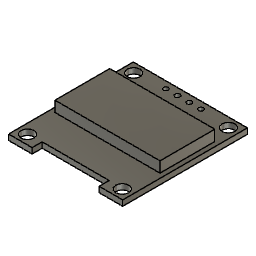
SSD1306 v2 (Autodesk Fusion 360 design; units mm, degrees)
Autodesk Fusion 360 part; units mm, degrees
note: some values were not read from the file. Set by a fixed rule: which sketch regions a step uses.
sketch "Sketch1" plane through (0, 0, 0) normal (0, 0, 1) x (1, 0, 0)
  line L0 (-12.35, 13.5) -> (12.35, 13.5)
  line L1 (12.35, 13.5) -> (12.35, -13.5)
  line L2 (-12.35, -13.5) -> (-12.35, 13.5)
  line L3 (0, 13.5) -> (0, -13.5)
  line L4 (-12.35, 0) -> (12.35, 0)
  circle A0 centre (-10.25, 11.5) radius 1.4
  circle A1 centre (10.25, 11.5) radius 1.4
  circle A2 centre (-10.25, -11.5) radius 1.4
  circle A3 centre (10.25, -11.5) radius 1.4
  line L5 (-7.2537, -13.5) -> (-7.2537, -11.3301)
  line L6 (-7.2537, -11.3301) -> (7.2537, -11.3301)
  line L7 (7.2537, -11.3301) -> (7.2537, -13.5)
  line L8 (7.2537, -13.5) -> (12.35, -13.5)
  line L9 (-12.35, -13.5) -> (-7.2537, -13.5)
  dimension "d1" = 24.7
  dimension "d2" = 27
  dimension "d11" = 2.8
  dimension "d12" = 2
  dimension "d13" = 2.1
  dimension "d15" = 23
  constraint horizontal L0
  constraint vertical L1
  constraint vertical L2
  constraint midpoint L0 L3.start
  constraint midpoint L2 L4.start
  constraint midpoint L1 L4.end
  constraint midpoint L4 origin
  constraint symmetric L3 A0 A1
  constraint symmetric L3 A2 A3
  constraint equal A0 A2
  constraint vertical A0.centre A2.centre
  constraint perpendicular L3 L6
  constraint symmetric L3 L5 L7
  constraint perpendicular L1 L8
  constraint perpendicular L5 L9
  measures "d1" distance of L0.start L0.end
  measures "d2" distance of L0.end L1.end
  measures "d11" diameter of A1
  measures "d12" distance of L0 A0.centre
  measures "d13" distance of L2 A0.centre
  measures "d15" distance of A0.centre A2.centre
extrude "Extrude2" add sketch "Sketch1" along normal blind 1.2 makes body 1
sketch "Sketch3" plane through (0, 0, 1.2) normal (0, 0, 1) x (-1, 0, 0)
  circle A0 centre (10.25, -11.5) radius 1.4
  circle A1 centre (-10.25, -11.5) radius 1.4
  circle A2 centre (-10.25, 11.5) radius 1.4
  circle A3 centre (10.25, 11.5) radius 1.4
  line L0 (-12.35, 13.5) -> (-12.35, -13.5)
  line L1 (-12.35, -13.5) -> (12.35, -13.5)
  line L2 (12.35, -13.5) -> (12.35, 13.5)
  line L3 (11.37, -7.42) -> (-11.37, -7.42)
  line L4 (-11.37, -7.42) -> (-11.37, 4.44)
  line L5 (-11.37, 4.44) -> (11.37, 4.44)
  line L6 (11.37, 4.44) -> (11.37, -7.42)
  line L7 (0, -13.5) -> (0, 13.5)
  line L8 (12.35, -13.5) -> (-12.35, -13.5)
  line L9 (12.35, 13.5) -> (7.2537, 13.5)
  line L10 (7.2537, 13.5) -> (7.2537, 11.3301)
  line L11 (7.2537, 11.3301) -> (-7.2537, 11.3301)
  line L12 (-7.2537, 11.3301) -> (-7.2537, 13.5)
  line L13 (-7.2537, 13.5) -> (-12.35, 13.5)
  dimension "d18" = 22.74
  dimension "d19" = 11.86
  dimension "d20" = 6.08
  constraint horizontal L3
  constraint vertical L4
  constraint horizontal L5
  constraint vertical L6
  constraint symmetric L4 L6 L7
  measures "d18" distance of L3.start L3.end
  measures "d19" distance of L3.start L5.end
  measures "d20" distance of L3 L8
extrude "Extrude3" add sketch "Sketch3" along normal blind 2.3 separate body contours L3 L5 L6 L7 | L3 L4 L5 L7 makes body 2
sketch "Sketch4" plane through (0, 0, 1.2) normal (0, 0, 1) x (-1, 0, 0)
  circle A0 centre (10.25, -11.5) radius 1.4
  circle A1 centre (-10.25, -11.5) radius 1.4
  circle A2 centre (10.25, 11.5) radius 1.4
  circle A3 centre (-10.25, 11.5) radius 1.4
  line L0 (12.35, -13.5) -> (12.35, 13.5)
  line L1 (12.35, 13.5) -> (7.2537, 13.5)
  line L2 (7.2537, 13.5) -> (7.2537, 11.3301)
  line L3 (7.2537, 11.3301) -> (-7.2537, 11.3301)
  line L4 (-7.2537, 11.3301) -> (-7.2537, 13.5)
  line L5 (-7.2537, 13.5) -> (-12.35, 13.5)
  line L6 (-12.35, 13.5) -> (-12.35, -13.5)
  line L7 (-12.35, -13.5) -> (12.35, -13.5)
  line L8 (8.3994, -12) -> (-8.3994, -12) construction
  line L9 (12.35, -13.5) -> (-12.35, -13.5) construction
  line L10 (0, -13.5) -> (0, 13.5) construction
  dimension "d23" = 1.5
  constraint horizontal L8
  constraint symmetric L8.start L8.end L10
  measures "d23" distance of L8 L9
sketch "Sketch5" plane through (0, 0, 1.2) normal (0, 0, 1) x (1, 0, 0)
  circle A0 centre (-3.81, 12) radius 0.5291
  circle A1 centre (-1.27, 12) radius 0.5291
  circle A2 centre (1.27, 12) radius 0.5291
  circle A3 centre (3.81, 12) radius 0.5291
  line L0 (0, 13.5) -> (0, -13.5)
  line L1 (-8.3994, 12) -> (8.3994, 12)
  dimension "d29" = 2.54
  dimension "d30" = 2.54
  constraint symmetric A0 A3 L0
  constraint symmetric A1 A2 L0
  constraint equal A0 A1
  constraint coincident A1.centre L1
  constraint coincident A0.centre L1
  measures "d29" horizontal distance of A0.centre A1.centre
  measures "d30" distance of A1.centre A2.centre
extrude "Extrude4" cut sketch "Sketch5" against normal up to surface (1.2 mm away) bodies 1
sketch "Sketch2" plane through (0, 0, 1.2) normal (0, 0, 1) x (-1, 0, 0)
  line L0 (13, 14) -> (-11.7, 14)
  line L1 (-11.7, 14) -> (-11.7, -13)
  line L2 (-11.7, -13) -> (13, -13)
  line L3 (13, -13) -> (13, 14)
